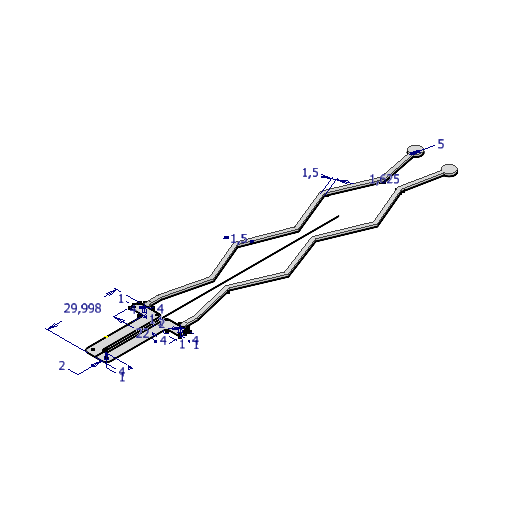
# Autodesk Inventor part: Part1
Saved by Autodesk Inventor 2025.4 (Build 294407000, 407)
## iProperties
Created: 2026-04-15
Part Number: Part1
Material: Generic
Document SubType Name: Modeling
Designer: gdira
Density: 1 g/cm^3
Appearance: Default
Author: gdira
Autodesk Inventor part; units mm, degrees
ref_plane "YZ Plane" through (0, 0, 0) normal (1, 0, 0) x (0, 1, 0)
ref_plane "XZ Plane" through (0, 0, 0) normal (0, 1, 0) x (-1, 0, 0)
ref_plane "XY Plane" through (0, 0, 0) normal (0, 0, 1) x (1, 0, 0)
sketch "Sketch1" plane through (0, 0, 0) normal (0, 1, 0) x (-1, 0, 0)
  line L0 (-7.6803, 9.5741) -> (-1.6803, 9.5741)
  line L1 (5.3197, -20.4249) -> (6.3252, -20.423)
  line L2 (-3.6803, -19.4275) -> (-3.6803, 4.5741)
  line L3 (-5.6803, 4.5741) -> (-5.6803, -19.4328)
  line L4 (0.3197, 7.5741) -> (0.3197, -12.405)
  line L5 (-6.6803, -20.4328) -> (-10.6803, -20.4328)
  line L6 (-9.6803, 7.5741) -> (-9.6803, -12.4328)
  arc A0 (-7.6803, 9.5741) -> (-9.6803, 7.5741) centre (-7.6803, 7.5741) ccw
  arc A1 (0.3197, 7.5741) -> (-1.6803, 9.5741) centre (-1.6803, 7.5741) ccw
  line L7 (6.3196, -19.425) -> (6.3196, -17.4232)
  line L8 (5.3196, -16.4232) -> (1.3197, -16.4232)
  line L9 (0.3197, -15.4232) -> (0.3197, -8.8508)
  line L10 (-15.6804, -19.4328) -> (-15.6804, -17.4328)
  line L11 (-14.6804, -16.4328) -> (-10.6803, -16.4328)
  line L12 (-9.6803, -15.4328) -> (-9.6803, -12.4328)
  arc A2 (-10.6803, -16.4328) -> (-9.6803, -15.4328) centre (-10.6803, -15.4328) ccw
  arc A3 (-14.6804, -16.4328) -> (-15.6804, -17.4328) centre (-14.6804, -17.4328) ccw
  arc A4 (-15.6804, -19.4328) -> (-14.6804, -20.4328) centre (-14.6804, -19.4328) ccw
  arc A5 (-6.6803, -20.4328) -> (-5.6803, -19.4328) centre (-6.6803, -19.4328) ccw
  arc A6 (5.3215, -20.425) -> (6.3196, -19.425) centre (5.3196, -19.425) ccw
  arc A7 (6.3196, -17.4232) -> (5.3196, -16.4232) centre (5.3196, -17.4232) ccw
  arc A8 (0.3197, -15.4232) -> (1.3197, -16.4232) centre (1.3197, -15.4232) ccw
  arc A9 (-4.6803, 5.5741) -> (-5.6803, 4.5741) centre (-4.6803, 4.5741) ccw
  arc A10 (-3.6803, 4.5741) -> (-4.6803, 5.5741) centre (-4.6803, 4.5741) ccw
  line L13 (3.8261, -22.4241) -> (3.8261, -26.4204)
  line L14 (2.3197, -26.4204) -> (2.3197, -21.9241)
  line L15 (3.8261, -26.4204) -> (-0.5079, -44.3248)
  line L16 (-2.0738, -44.418) -> (2.3602, -26.1006)
  line L17 (-2.0738, -44.418) -> (5.5193, -62.3259)
  line L18 (5.8312, -63.0856) -> (6.3886, -62.8493)
  line L19 (7.1246, -62.3259) -> (-0.5079, -44.3248)
  line L20 (7.1246, -62.3259) -> (-0.1739, -81.4204)
  line L21 (-1.5617, -80.8511) -> (5.817, -61.547)
  line L22 (3.326, -136.4319) -> (-0.1748, -118.6507)
  line L23 (7.5882, -100.3419) -> (-0.1748, -118.6507)
  line L24 (7.5882, -100.3419) -> (-0.1739, -81.4204)
  line L25 (-1.5617, -81.9897) -> (5.963, -100.3323)
  line L26 (-4.6803, 9.5741) -> (-4.6803, -95.9408)
  line L27 (5.8225, -20.4241) -> (4.8261, -20.4241)
  line L28 (-3.6803, -19.4241) -> (-3.6803, -19.0268)
  arc A11 (-3.6803, -19.4241) -> (-2.6803, -20.4241) centre (-2.6803, -19.4241) ccw
  line L29 (3.8261, -22.4241) -> (3.8261, -21.4241)
  line L30 (2.3197, -21.9241) -> (2.3197, -21.4241)
  arc A12 (4.8261, -20.4241) -> (3.8261, -21.4241) centre (4.8261, -21.4241) ccw
  line L31 (-2.6803, -20.4241) -> (1.3197, -20.4241)
  arc A13 (2.3197, -21.4241) -> (1.3197, -20.4241) centre (1.3197, -21.4241) ccw
  arc A14 (-10.6803, -20.4328) -> (-11.6803, -21.4328) centre (-10.6803, -21.4328) ccw
  line L32 (-14.1866, -20.4328) -> (-14.6804, -20.4328)
  arc A15 (-13.1866, -21.4328) -> (-14.1866, -20.4328) centre (-14.1866, -21.4328) ccw
  line L33 (-1.2422, -80.0152) -> (-1.7793, -81.4204)
  line L34 (-1.7793, -81.4204) -> (-1.4262, -82.32)
  line L35 (5.8225, -20.4241) -> (-1.7793, -20.4241)
  line L36 (-7.6952, -20.4328) -> (-14.6804, -20.4328)
  line L37 (7.1246, -62.3259) -> (5.5193, -62.3259)
  line L38 (3.326, -136.4319) -> (1.826, -136.4319)
  arc A16 (1.4006, -134.2255) -> (2.8365, -133.9455) centre (2.576, -136.4319) ccw
  line L39 (-1.7998, -118.6507) -> (1.4006, -134.2255)
  line L40 (-1.8041, -118.6507) -> (5.963, -100.3323)
  line L41 (-1.7731, -118.7808) -> (-1.8012, -118.6439)
  line L42 (-13.1866, -22.4241) -> (-13.1866, -26.4204)
  line L43 (-11.6803, -26.4204) -> (-11.6803, -21.9241)
  line L44 (-13.1866, -26.4204) -> (-8.8527, -44.3248)
  line L45 (-7.2868, -44.418) -> (-11.7208, -26.1006)
  line L46 (-7.2868, -44.418) -> (-14.8799, -62.3259)
  line L47 (-15.1918, -63.0856) -> (-15.7492, -62.8493)
  line L48 (-16.4852, -62.3259) -> (-8.8527, -44.3248)
  line L49 (-16.4852, -62.3259) -> (-9.1866, -81.4204)
  line L50 (-7.7989, -80.8511) -> (-15.1776, -61.547)
  line L51 (-12.6866, -136.4319) -> (-9.1858, -118.6507)
  line L52 (-7.7989, -81.9897) -> (-15.3236, -100.3323)
  line L53 (-16.9488, -100.3419) -> (-9.1866, -81.4204)
  line L54 (-16.9488, -100.3419) -> (-9.1858, -118.6507)
  line L55 (-13.1866, -22.4241) -> (-13.1866, -21.4241)
  line L56 (-11.6803, -21.9241) -> (-11.6803, -21.4241)
  arc A17 (-13.1866, -21.4241) -> (-14.1866, -20.4241) centre (-14.1866, -21.4241) ccw
  arc A18 (-10.6803, -20.4241) -> (-11.6803, -21.4241) centre (-10.6803, -21.4241) ccw
  line L57 (-8.1184, -80.0152) -> (-7.5813, -81.4204)
  line L58 (-7.5813, -81.4204) -> (-7.9344, -82.32)
  line L59 (-16.4852, -62.3259) -> (-14.8799, -62.3259)
  line L60 (-12.6866, -136.4319) -> (-11.1866, -136.4319)
  arc A19 (-12.1971, -133.9455) -> (-10.7612, -134.2255) centre (-11.9366, -136.4319) ccw
  line L61 (-7.5608, -118.6507) -> (-10.7612, -134.2255)
  line L62 (-7.5565, -118.6507) -> (-15.3236, -100.3323)
  line L63 (-7.5875, -118.7808) -> (-7.5594, -118.6439)
  point P0 (0, 0)
  point P1 (0.3141, -20.4341)
  point P2 (-15.6804, -20.4328)
  point P3 (5.8225, -20.4239)
  point P4 (6.3196, -16.4232)
  point P5 (-15.6804, -16.4328)
  point P6 (-4.6803, 5.5741)
  point P7 (-15.6804, -18.4328)
  point P8 (6.3196, -18.4241)
  point P9 (-0.2865, -43.5467)
  point P10 (-0.1738, -118.0871)
  point P11 (-1.6654, -118.3237)
  point P12 (-0.2865, -119.2942)
  point P13 (5.8172, -101.2939)
  point P14 (2.3197, -26.2677)
  point P15 (2.3197, -20.4241)
  point P16 (-13.1866, -20.4328)
  point P17 (5.7375, -20.4241)
  point P18 (5.3626, -20.4241)
  point P19 (5.3391, -20.4248)
  point P20 (-3.6803, -19.4241)
  point P21 (-9.0741, -43.5467)
  point P22 (-9.0741, -119.2942)
  point P23 (-9.1868, -118.0871)
  point P24 (-7.6952, -118.3237)
  point P25 (-15.1778, -101.2939)
  point P26 (-11.6803, -26.2677)
  point P27 (-10.812, -20.4328)
  point P28 (-14.0549, -20.4328)
  dimension "d2" = 4
  dimension "d3" = 4
  dimension "d4" = 2
  dimension "d5" = 4
  dimension "d6" = 29.998
  dimension "d7" = 2
  dimension "d9" = 4
  dimension "d10" = 1
  dimension "d11" = 1
  dimension "d14" = 22
  dimension "d39" = 1.5
  dimension "d49" = 1
  dimension "d50" = 1
  dimension "d51" = 1
  dimension "d52" = 1
  dimension "d54" = 1.5
  dimension "d56" = 4
  dimension "d59" = 5
  dimension "d107" = 1.625
  constraints: 128 end point, 41 symmetric about line, 40 point on circle, 36 point on line, 27 tangent, 20 centre point, 8 equal radius, 7 parallel, 6 horizontal, 6 perpendicular, 5 midpoint, 5 vertical, 1 collinear, 9 other
  measures "d2" distance between parallel lines of L2 L4
  measures "d3" distance between parallel lines of L6 L3
  measures "d4" distance between parallel lines of L3 L2
  measures "d5" distance of L26.start point (-4.68, 5.574)
  measures "d6" distance from line of point (5.822, -20.424) L0
  measures "d7" radius of A0
  measures "d9" distance of point (-15.68, -20.433) point (-15.68, -16.433)
  measures "d10" radius of A2
  measures "d11" radius of A9
  measures "d14" distance of point (-15.68, -18.433) point (6.32, -18.424)
  measures "d39" distance of L19.start L18.start
  measures "d49" radius of A12
  measures "d50" radius of A13
  measures "d51" radius of A14
  measures "d52" radius of A15
  measures "d54" distance between parallel lines of L25 L24
  measures "d56" distance of L31.start L31.end
  measures "d59" diameter of A16
  measures "d107" distance of L22.end L39.start
extrude "Extrusion1" add sketch "Sketch1" along normal blind 0.15 contours L0 L26 A9 L3 A5 L5 L36 L32 A4 L10 A3 L11 A2 L12 L6 A0 | L0 A1 L4 L9 A8 L8 A7 L7 A6 L27 L35 L31 A11 L2 A10 L26
extrude "Extrusion2" add sketch "Sketch1" along normal blind 1 contours A14 L56 L43 L45 L46 L59 L48 L44 L42 L55 A15 A17 L36 A18 | L35 A12 L29 L13 L15 L19 L37 L17 L16 L14 L30 A13 | L50 L57 L58 L52 L62 L63 L61 A19 L51 L54 L53 L49 L59 | L37 L20 L24 L23 L22 A16 L39 L41 L40 L25 L34 L33 L21
fillet "Fillet1" radius 2 2 edges at (-3.0729, 1, -20.4241) (12.4335, 1, -20.4328)
body "Solid1"
